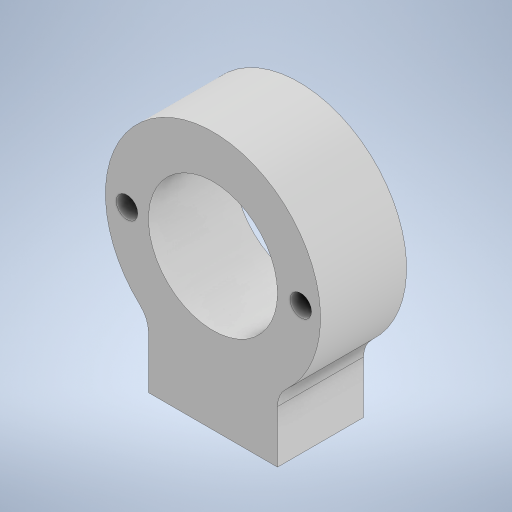
# Autodesk Inventor part: TPS base
Saved by Autodesk Inventor 2023 (Build 270158000, 158)
## iProperties
Created: 2023-07-25
Part Number: TPS base
Material: Generic
Document SubType Name: Modeling
Designer: User
Density: 1 g/cm^3
Appearance: Default
Author: User
Autodesk Inventor part; units mm, degrees
ref_plane "YZ Plane" through (0, 0, 0) normal (1, 0, 0) x (0, 1, 0)
ref_plane "XZ Plane" through (0, 0, 0) normal (0, 1, 0) x (-1, 0, 0)
ref_plane "XY Plane" through (0, 0, 0) normal (0, 0, 1) x (1, 0, 0)
sketch "Sketch1" plane through (0, 0, 0) normal (0, 0, 1) x (1, 0, 0)
  circle A0 centre (0, 0) radius 15
  arc A1 (15, -20) -> (-15, -20) centre (0, 0) ccw
  line L0 (-15, -20) -> (-15, -35)
  line L1 (-15, -35) -> (15, -35)
  line L2 (15, -20) -> (15, -35)
  dimension "d0" = 30
  dimension "d1" = 50
  dimension "d2" = 15
  constraints: 6 end point, 2 centre point, 2 coincident, 2 perpendicular, 2 point on circle, 2 tangent, 1 vertical
  measures "d0" diameter of A0
  measures "d1" diameter of A1
  measures "d2" distance from line of L0.start L1
extrude "Extrusion1" add sketch "Sketch1" along normal blind 20
sketch "Sketch2" plane through (0, 0, 20) normal (0, 0, 1) x (1, 0, 0)
  point P0 (0, 0)
  point P1 (-19.9785, -0.185)
  point P2 (20.4097, 0.2462)
hole "Hole1" at (0, 0, 20) at (-19.9785, -0.185, 20) at (20.4097, 0.2462, 20) direction (0, 0, -1) diameter 5 end through all
fillet "Fillet1" radius 6 2 edges at (15, -20, 10) (-15, -20, 10)
body "Solid1"
